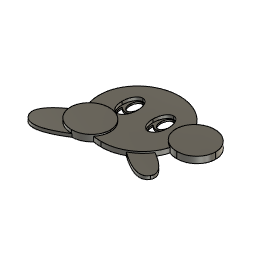
Kirby (Autodesk Fusion 360 design; units mm, degrees)
Autodesk Fusion 360 part; units mm, degrees
note: some values were not read from the file. Set by a fixed rule: which sketch regions a step uses.
sketch "Body" plane through (0, 0, 0) normal (0, 0, 1) x (1, 0, 0)
  spline S0 degree 2 poles (-25.3043, -9.4119) (-88.3517, -41.3968) (-76.8327, -61.1714) knots 0 0 0 1 1 1
  spline S1 degree 2 poles (-76.8327, -61.1714) (-65.3132, -80.9459) (-14.8426, -44.1924) knots 0 0 0 1 1 1
  spline S2 degree 3 poles (-14.8426, -44.1924) (-14.5009, -28.664) (-10.0033, -8.8636) (-25.3043, -9.4119) knots 0 0 0 0 1 1 1 1
  line L0 (-25.3043, -9.4119) -> (-25.3043, -9.4119)
  spline S3 degree 2 poles (-25.3043, -9.4119) (-88.3517, -41.3968) (-76.8327, -61.1714) knots 0 0 0 1 1 1
  spline S4 degree 2 poles (-76.8327, -61.1714) (-65.3132, -80.9459) (-14.8426, -44.1924) knots 0 0 0 1 1 1
  spline S5 degree 3 poles (-14.8426, -44.1924) (-14.5009, -28.664) (-10.0033, -8.8636) (-25.3043, -9.4119) knots 0 0 0 0 1 1 1 1
  line L1 (-25.3043, -9.4119) -> (-25.3043, -9.4119)
  spline S6 degree 3 poles (50.1135, 2.3188) (50.1135, -24.7089) (27.1933, -46.6187) (-1.0791, -46.6187) knots 0 0 0 0 1 1 1 1
  spline S7 degree 3 poles (-1.0791, -46.6187) (-29.3524, -46.6187) (-52.2718, -24.7089) (-52.2718, 2.3188) knots 0 0 0 0 1 1 1 1
  spline S8 degree 3 poles (-52.2718, 2.3188) (-52.2718, 29.3466) (-29.3516, 51.2564) (-1.0791, 51.2564) knots 0 0 0 0 1 1 1 1
  spline S9 degree 3 poles (-1.0791, 51.2564) (27.1941, 51.2564) (50.1135, 29.3466) (50.1135, 2.3188) knots 0 0 0 0 1 1 1 1
  spline S10 degree 3 poles (50.1135, 2.3188) (50.1135, -24.7089) (27.1933, -46.6187) (-1.0791, -46.6187) knots 0 0 0 0 1 1 1 1
  spline S11 degree 3 poles (-1.0791, -46.6187) (-29.3524, -46.6187) (-52.2718, -24.7089) (-52.2718, 2.3188) knots 0 0 0 0 1 1 1 1
  spline S12 degree 3 poles (-52.2718, 2.3188) (-52.2718, 29.3466) (-29.3516, 51.2564) (-1.0791, 51.2564) knots 0 0 0 0 1 1 1 1
  spline S13 degree 3 poles (-1.0791, 51.2564) (27.1941, 51.2564) (50.1135, 29.3466) (50.1135, 2.3188) knots 0 0 0 0 1 1 1 1
  spline S14 degree 3 poles (50.1135, 2.3188) (50.1135, -24.7089) (27.1933, -46.6187) (-1.0791, -46.6187) knots 0 0 0 0 1 1 1 1
  spline S15 degree 3 poles (-1.0791, -46.6187) (-29.3524, -46.6187) (-52.2718, -24.7089) (-52.2718, 2.3188) knots 0 0 0 0 1 1 1 1
  spline S16 degree 3 poles (-52.2718, 2.3188) (-52.2718, 29.3466) (-29.3516, 51.2564) (-1.0791, 51.2564) knots 0 0 0 0 1 1 1 1
  spline S17 degree 3 poles (-1.0791, 51.2564) (27.1941, 51.2564) (50.1135, 29.3466) (50.1135, 2.3188) knots 0 0 0 0 1 1 1 1
  spline S18 degree 3 poles (26.4728, 9.9863) (26.4728, 1.0187) (22.1358, -6.2511) (16.7858, -6.2511) knots 0 0 0 0 1 1 1 1
  spline S19 degree 3 poles (16.7858, -6.2511) (11.4358, -6.2511) (7.0988, 1.0187) (7.0988, 9.9863) knots 0 0 0 0 1 1 1 1
  spline S20 degree 3 poles (7.0988, 9.9863) (7.0988, 18.9539) (11.4358, 26.2237) (16.7858, 26.2237) knots 0 0 0 0 1 1 1 1
  spline S21 degree 3 poles (16.7858, 26.2237) (22.1358, 26.2237) (26.4728, 18.9539) (26.4728, 9.9863) knots 0 0 0 0 1 1 1 1
  spline S22 degree 3 poles (22.4193, 15.7063) (22.4193, 10.4907) (19.8969, 6.2626) (16.7853, 6.2626) knots 0 0 0 0 1 1 1 1
  spline S23 degree 3 poles (16.7853, 6.2626) (13.6738, 6.2626) (11.1514, 10.4907) (11.1514, 15.7063) knots 0 0 0 0 1 1 1 1
  spline S24 degree 3 poles (11.1514, 15.7063) (11.1514, 20.9218) (13.6738, 25.1499) (16.7853, 25.1499) knots 0 0 0 0 1 1 1 1
  spline S25 degree 3 poles (16.7853, 25.1499) (19.8969, 25.1499) (22.4193, 20.9218) (22.4193, 15.7063) knots 0 0 0 0 1 1 1 1
  spline S26 degree 3 poles (9.5098, 7.6408) (17.882, 0.7681) (20.4581, 5.1787) (23.5114, 7.6408) knots 0 0 0 0 1 1 1 1
  spline S27 degree 3 poles (23.5114, 7.6408) (23.149, 3.5887) (24.7202, -1.2015) (17.4707, -5.2533) knots 0 0 0 0 1 1 1 1
  spline S28 degree 3 poles (17.4707, -5.2533) (9.8696, -2.4809) (9.2832, 2.7921) (9.5099, 7.6408) knots 0 0 0 0 1 1 1 1
  line L2 (9.5099, 7.6408) -> (9.5098, 7.6408)
  spline S29 degree 3 poles (-11.9676, 9.9863) (-11.9676, 1.0187) (-16.3046, -6.2511) (-21.6547, -6.2511) knots 0 0 0 0 1 1 1 1
  spline S30 degree 3 poles (-21.6547, -6.2511) (-27.0047, -6.2511) (-31.3417, 1.0187) (-31.3417, 9.9863) knots 0 0 0 0 1 1 1 1
  spline S31 degree 3 poles (-31.3417, 9.9863) (-31.3417, 18.9539) (-27.0047, 26.2237) (-21.6547, 26.2237) knots 0 0 0 0 1 1 1 1
  spline S32 degree 3 poles (-21.6547, 26.2237) (-16.3046, 26.2237) (-11.9676, 18.9539) (-11.9676, 9.9863) knots 0 0 0 0 1 1 1 1
  spline S33 degree 3 poles (-16.0211, 15.7063) (-16.0211, 10.4907) (-18.5435, 6.2626) (-21.6551, 6.2626) knots 0 0 0 0 1 1 1 1
  spline S34 degree 3 poles (-21.6551, 6.2626) (-24.7667, 6.2626) (-27.2891, 10.4907) (-27.2891, 15.7063) knots 0 0 0 0 1 1 1 1
  spline S35 degree 3 poles (-27.2891, 15.7063) (-27.2891, 20.9218) (-24.7667, 25.1499) (-21.6551, 25.1499) knots 0 0 0 0 1 1 1 1
  spline S36 degree 3 poles (-21.6551, 25.1499) (-18.5435, 25.1499) (-16.0211, 20.9218) (-16.0211, 15.7063) knots 0 0 0 0 1 1 1 1
  spline S37 degree 3 poles (-28.9306, 7.6408) (-20.5585, 0.7681) (-17.9824, 5.1787) (-14.929, 7.6408) knots 0 0 0 0 1 1 1 1
  spline S38 degree 3 poles (-14.929, 7.6408) (-15.2915, 3.5887) (-13.7203, -1.2015) (-20.9698, -5.2533) knots 0 0 0 0 1 1 1 1
  spline S39 degree 3 poles (-20.9698, -5.2533) (-28.5709, -2.4809) (-29.1573, 2.7921) (-28.9306, 7.6408) knots 0 0 0 0 1 1 1 1
  line L3 (-28.9306, 7.6408) -> (-28.9306, 7.6408)
  spline S40 degree 3 poles (83.6748, 11.5654) (83.6748, -1.5125) (72.5844, -12.114) (58.9042, -12.114) knots 0 0 0 0 1 1 1 1
  spline S41 degree 3 poles (58.9042, -12.114) (45.2236, -12.114) (34.1337, -1.5125) (34.1337, 11.5654) knots 0 0 0 0 1 1 1 1
  spline S42 degree 3 poles (34.1337, 11.5654) (34.1337, 24.6433) (45.224, 35.2448) (58.9042, 35.2448) knots 0 0 0 0 1 1 1 1
  spline S43 degree 3 poles (58.9042, 35.2448) (72.5848, 35.2448) (83.6748, 24.6433) (83.6748, 11.5654) knots 0 0 0 0 1 1 1 1
  spline S44 degree 3 poles (83.6748, 11.5654) (83.6748, -1.5125) (72.5844, -12.114) (58.9042, -12.114) knots 0 0 0 0 1 1 1 1
  spline S45 degree 3 poles (58.9042, -12.114) (45.2236, -12.114) (34.1337, -1.5125) (34.1337, 11.5654) knots 0 0 0 0 1 1 1 1
  spline S46 degree 3 poles (34.1337, 11.5654) (34.1337, 24.6433) (45.224, 35.2448) (58.9042, 35.2448) knots 0 0 0 0 1 1 1 1
  spline S47 degree 3 poles (58.9042, 35.2448) (72.5848, 35.2448) (83.6748, 24.6433) (83.6748, 11.5654) knots 0 0 0 0 1 1 1 1
  spline S48 degree 3 poles (83.6748, 11.5654) (83.6748, -1.5125) (72.5844, -12.114) (58.9042, -12.114) knots 0 0 0 0 1 1 1 1
  spline S49 degree 3 poles (58.9042, -12.114) (45.2236, -12.114) (34.1337, -1.5125) (34.1337, 11.5654) knots 0 0 0 0 1 1 1 1
  spline S50 degree 3 poles (34.1337, 11.5654) (34.1337, 24.6433) (45.224, 35.2448) (58.9042, 35.2448) knots 0 0 0 0 1 1 1 1
  spline S51 degree 3 poles (58.9042, 35.2448) (72.5848, 35.2448) (83.6748, 24.6433) (83.6748, 11.5654) knots 0 0 0 0 1 1 1 1
  spline S52 degree 3 poles (-5.6275, -30.6069) (-5.6275, -43.6848) (-16.7179, -54.2863) (-30.3981, -54.2863) knots 0 0 0 0 1 1 1 1
  spline S53 degree 3 poles (-30.3981, -54.2863) (-44.0787, -54.2863) (-55.1687, -43.6848) (-55.1687, -30.6069) knots 0 0 0 0 1 1 1 1
  spline S54 degree 3 poles (-55.1687, -30.6069) (-55.1687, -17.529) (-44.0783, -6.9275) (-30.3981, -6.9275) knots 0 0 0 0 1 1 1 1
  spline S55 degree 3 poles (-30.3981, -6.9275) (-16.7175, -6.9275) (-5.6275, -17.529) (-5.6275, -30.6069) knots 0 0 0 0 1 1 1 1
  spline S56 degree 3 poles (-5.6275, -30.6069) (-5.6275, -43.6848) (-16.7179, -54.2863) (-30.3981, -54.2863) knots 0 0 0 0 1 1 1 1
  spline S57 degree 3 poles (-30.3981, -54.2863) (-44.0787, -54.2863) (-55.1687, -43.6848) (-55.1687, -30.6069) knots 0 0 0 0 1 1 1 1
  spline S58 degree 3 poles (-55.1687, -30.6069) (-55.1687, -17.529) (-44.0783, -6.9275) (-30.3981, -6.9275) knots 0 0 0 0 1 1 1 1
  spline S59 degree 3 poles (-30.3981, -6.9275) (-16.7175, -6.9275) (-5.6275, -17.529) (-5.6275, -30.6069) knots 0 0 0 0 1 1 1 1
  spline S60 degree 3 poles (-5.6275, -30.6069) (-5.6275, -43.6848) (-16.7179, -54.2863) (-30.3981, -54.2863) knots 0 0 0 0 1 1 1 1
  spline S61 degree 3 poles (-30.3981, -54.2863) (-44.0787, -54.2863) (-55.1687, -43.6848) (-55.1687, -30.6069) knots 0 0 0 0 1 1 1 1
  spline S62 degree 3 poles (-55.1687, -30.6069) (-55.1687, -17.529) (-44.0783, -6.9275) (-30.3981, -6.9275) knots 0 0 0 0 1 1 1 1
  spline S63 degree 3 poles (-30.3981, -6.9275) (-16.7175, -6.9275) (-5.6275, -17.529) (-5.6275, -30.6069) knots 0 0 0 0 1 1 1 1
  spline S64 degree 2 poles (30.1659, -16.2031) (72.4206, -37.6387) (64.7005, -50.8914) knots 0 0 0 1 1 1
  spline S65 degree 2 poles (64.7005, -50.8914) (56.98, -64.144) (23.1543, -39.5125) knots 0 0 0 1 1 1
  spline S66 degree 3 poles (23.1543, -39.5125) (22.9254, -29.1056) (19.9111, -15.8357) (30.1658, -16.2031) knots 0 0 0 0 1 1 1 1
  line L4 (30.1658, -16.2031) -> (30.1659, -16.2031)
  spline S67 degree 2 poles (30.1659, -16.2031) (72.4206, -37.6387) (64.7005, -50.8914) knots 0 0 0 1 1 1
  spline S68 degree 2 poles (64.7005, -50.8914) (56.98, -64.144) (23.1543, -39.5125) knots 0 0 0 1 1 1
  spline S69 degree 3 poles (23.1543, -39.5125) (22.9254, -29.1056) (19.9111, -15.8357) (30.1658, -16.2031) knots 0 0 0 0 1 1 1 1
  line L5 (30.1658, -16.2031) -> (30.1659, -16.2031)
  spline S70 degree 2 poles (-5.8174, -15.9483) (11.0968, -19.7821) (12.6755, -17.3014) knots 0 0 0 1 1 1
  spline S71 degree 2 poles (12.6755, -17.3014) (14.2541, -14.8207) (14.2541, -15.0463) knots 0 0 0 1 1 1
  spline S72 degree 2 poles (-5.8174, -15.9483) (11.0968, -19.7821) (12.6755, -17.3014) knots 0 0 0 1 1 1
  spline S73 degree 2 poles (12.6755, -17.3014) (14.2541, -14.8207) (14.2541, -15.0463) knots 0 0 0 1 1 1
  spline S74 degree 2 poles (-5.8174, -15.9483) (11.0968, -19.7821) (12.6755, -17.3014) knots 0 0 0 1 1 1
  spline S75 degree 2 poles (12.6755, -17.3014) (14.2541, -14.8207) (14.2541, -15.0463) knots 0 0 0 1 1 1
  spline S76 degree 2 poles (-5.8174, -15.9483) (11.0968, -19.7821) (12.6755, -17.3014) knots 0 0 0 1 1 1
  spline S77 degree 2 poles (12.6755, -17.3014) (14.2541, -14.8207) (14.2541, -15.0463) knots 0 0 0 1 1 1
  spline S78 degree 2 poles (-5.8174, -15.9483) (11.0968, -19.7821) (12.6755, -17.3014) knots 0 0 0 1 1 1
  spline S79 degree 2 poles (12.6755, -17.3014) (14.2541, -14.8207) (14.2541, -15.0463) knots 0 0 0 1 1 1
  spline S80 degree 2 poles (-5.8174, -15.9483) (11.0968, -19.7821) (12.6755, -17.3014) knots 0 0 0 1 1 1
  spline S81 degree 2 poles (12.6755, -17.3014) (14.2541, -14.8207) (14.2541, -15.0463) knots 0 0 0 1 1 1
  spline S82 degree 2 poles (-5.8174, -15.9483) (11.0968, -19.7821) (12.6755, -17.3014) knots 0 0 0 1 1 1
  spline S83 degree 2 poles (12.6755, -17.3014) (14.2541, -14.8207) (14.2541, -15.0463) knots 0 0 0 1 1 1
  spline S84 degree 2 poles (-5.8174, -15.9483) (11.0968, -19.7821) (12.6755, -17.3014) knots 0 0 0 1 1 1
  spline S85 degree 2 poles (12.6755, -17.3014) (14.2541, -14.8207) (14.2541, -15.0463) knots 0 0 0 1 1 1
extrude "Extrude1" add sketch "Body" along normal blind 6 contours S0 S1 S2 S3 S4 S5 S7 S11 S15 | S0 S1 S2 S3 S4 S5 S7 S11 S15 S52 S54 S55 S56 S58 S59 S60 S62 S63 | S6 S7 S8 S9 S10 S11 S12 S13 S14 S15 S16 S17 S41 S42 S45 S46 S49 S50 S52 S54 S55 S56 S58 S59 S60 S62 S63 S64 S65 S66 S67 S68 S69 | S6 S10 S14 S64 S65 S66 S67 S68 S69 | S6 S9 S10 S13 S14 S17 S41 S42 S45 S46 S49 S50
extrude "Extrude2" add sketch "Body" along normal blind 8 contours S0 S1 S2 S3 S4 S5 S7 S11 S15 | S0 S1 S2 S3 S4 S5 S7 S11 S15 S52 S54 S55 S56 S58 S59 S60 S62 S63 | S0 S1 S3 S4 S7 S11 S15 S52 S53 S54 S56 S57 S58 S60 S61 S62 | S0 S3 S7 S11 S15 S54 S58 S62 | S1 S4 S7 S11 S15 S52 S56 S60 | S6 S9 S10 S13 S14 S17 S40 S41 S42 S43 S44 S45 S46 S47 S48 S49 S50 S51 | S6 S9 S10 S13 S14 S17 S41 S42 S45 S46 S49 S50
extrude "Extrude3" add sketch "Body" along normal blind 4 contours S0 S1 S2 S3 S4 S5 S7 S11 S15 | S0 S1 S3 S4 S7 S11 S15 S52 S53 S54 S56 S57 S58 S60 S61 S62 | S0 S1 S3 S4 S52 S53 S54 S56 S57 S58 S60 S61 S62 | S6 S10 S14 S64 S65 S66 S67 S68 S69 | S6 S10 S14 S64 S65 S67 S68
extrude "Extrude4" add sketch "Body" along normal blind 2 contours S18 S19 S20 S21 | S29 S30 S31 S32
named bodies: "Kirby_Keychain"
